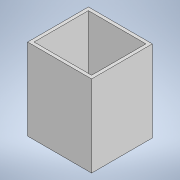
# Autodesk Inventor part: Крышка USB
Saved by Autodesk Inventor 2020 (Build 240168000, 168)
## iProperties
Created: 2021-06-28
Part Number: Крышка USB
Material: Типовые
Document SubType Name: Modeling
Designer: Антон
Density: 1 g/cm^3
Appearance: По умолчанию
Author: Антон
Autodesk Inventor part; units mm, degrees
ref_plane "YZ Plane" through (0, 0, 0) normal (1, 0, 0) x (0, 1, 0)
ref_plane "XZ Plane" through (0, 0, 0) normal (0, 1, 0) x (-1, 0, 0)
ref_plane "XY Plane" through (0, 0, 0) normal (0, 0, 1) x (1, 0, 0)
sketch "Эскиз1" plane through (0, 0, 0) normal (0, 1, 0) x (-1, 0, 0)
  line L0 (0, 0) -> (20, 0)
  line L1 (20, 0) -> (20, -19)
  line L2 (20, -19) -> (0, -19)
  line L3 (0, -19) -> (0, 0)
  dimension "d0" = 20
  dimension "d1" = 19
  constraints: 8 end point, 2 parallel, 1 horizontal, 1 perpendicular
  measures "d0" distance of L1.end L2.end
  measures "d1" distance of L0.end L1.end
extrude "Выдавливание1" add sketch "Эскиз1" along normal blind 25.5
sketch "Эскиз2" plane through (0, 25.5, 0) normal (0, 1, 0) x (1, 0, 0)
  line L0 (-1, 1) -> (-19, 1)
  line L1 (-19, 1) -> (-19, 18)
  line L2 (-19, 18) -> (-1, 18)
  line L3 (-1, 18) -> (-1, 1)
  line L4 (-20, 0) -> (0, 0) projected
  line L5 (0, 0) -> (0, 19) projected
  line L6 (0, 19) -> (-20, 19) projected
  line L7 (-20, 19) -> (-20, 0) projected
  dimension "d4" = 1
  dimension "d5" = 1
  dimension "d6" = 1
  dimension "d7" = 1
  constraints: 8 end point, 2 parallel, 1 horizontal, 1 perpendicular
  measures "d4" distance between parallel lines of L4 L0
  measures "d5" distance between parallel lines of L5 L3
  measures "d6" distance between parallel lines of L6 L2
  measures "d7" distance between parallel lines of L7 L1
extrude "Выдавливание2" cut sketch "Эскиз2" against normal blind 24.5 contours L0 L1 L2 L3
